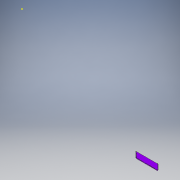
# Autodesk Inventor part: BaseBandAmp_Top_SolderMaskLower
Saved by Autodesk Inventor 2018 (Build 220112000, 112)
## iProperties
Created: 2018-03-29
Part Number: BaseBandAmp_Top_SolderMaskLower
Material: Generic
Document SubType Name: Modeling
Designer: Eric Weeks
Density: 1 g/cm^3
Appearance: Default
Author: Eric Weeks
Autodesk Inventor part; units mm, degrees
ref_plane "YZ Plane" through (0, 0, 0) normal (1, 0, 0) x (0, 1, 0)
ref_plane "XZ Plane" through (0, 0, 0) normal (0, 1, 0) x (-1, 0, 0)
ref_plane "XY Plane" through (0, 0, 0) normal (0, 0, 1) x (1, 0, 0)
sketch "Sketch1" plane through (0, 0, 0) normal (0, 0, 1) x (1, 0, 0)
  circle A0 centre (3267.7354, -2038.7056) radius 4.8387 projected
  circle A1 centre (3267.7354, -2038.7056) radius 4.8387 projected
  circle A2 centre (3287.0902, -2038.7056) radius 4.8387 projected
  circle A3 centre (3287.0902, -2038.7056) radius 4.8387 projected
  circle A4 centre (3306.445, -2038.7056) radius 4.8387 projected
  circle A5 centre (3306.445, -2038.7056) radius 4.8387 projected
  circle A6 centre (3325.7998, -2038.7056) radius 4.8387 projected
  circle A7 centre (3325.7998, -2038.7056) radius 4.8387 projected
  circle A8 centre (3345.1546, -2038.7056) radius 4.8387 projected
  circle A9 centre (3345.1546, -2038.7056) radius 4.8387 projected
  circle A10 centre (3364.5094, -2038.7056) radius 4.8387 projected
  circle A11 centre (3364.5094, -2038.7056) radius 4.8387 projected
  circle A12 centre (3383.8642, -2038.7056) radius 4.8387 projected
  circle A13 centre (3383.8642, -2038.7056) radius 4.8387 projected
  line L0 (3864.5338, -2031.6901) -> (3864.5338, -2031.8324) projected
  line L1 (3864.5338, -2031.8324) -> (3862.959, -2040.7808) projected
  line L2 (3862.959, -2040.7808) -> (3862.7558, -2041.3066) projected
  line L3 (3862.7558, -2041.3066) -> (3858.5648, -2048.5583) projected
  line L4 (3858.5648, -2048.5583) -> (3858.2092, -2048.9875) projected
  line L5 (3858.2092, -2048.9875) -> (3851.783, -2054.3698) projected
  line L6 (3851.783, -2054.3698) -> (3851.5544, -2054.5146) projected
  line L7 (3851.5544, -2054.5146) -> (3851.3004, -2054.6492) projected
  line L8 (3851.3004, -2054.6492) -> (3843.0962, -2057.6362) projected
  line L9 (3843.0962, -2057.6362) -> (3842.893, -2057.6718) projected
  line L10 (3842.893, -2057.6718) -> (3842.6898, -2057.7277) projected
  line L11 (3842.6898, -2057.7277) -> (3838.4988, -2058.096) projected
  line L12 (3838.4988, -2058.096) -> (3838.4226, -2058.0883) projected
  line L13 (3838.4226, -2058.0883) -> (3838.3464, -2058.101) projected
  line L14 (3838.3464, -2058.101) -> (3258.7692, -2058.101) projected
  line L15 (3258.7692, -2058.101) -> (3258.6168, -2058.0756) projected
  line L16 (3258.6168, -2058.0756) -> (3258.4898, -2058.0756) projected
  line L17 (3258.4898, -2058.0756) -> (3249.5236, -2056.4983) projected
  line L18 (3249.5236, -2056.4983) -> (3249.4982, -2056.4881) projected
  line L19 (3249.4982, -2056.4881) -> (3249.0156, -2056.3078) projected
  line L20 (3249.0156, -2056.3078) -> (3241.7512, -2052.1193) projected
  line L21 (3241.7512, -2052.1193) -> (3241.3194, -2051.7612) projected
  line L22 (3241.3194, -2051.7612) -> (3235.9346, -2045.3452) projected
  line L23 (3235.9346, -2045.3452) -> (3235.7568, -2045.0378) projected
  line L24 (3235.7568, -2045.0378) -> (3235.6552, -2044.86) projected
  line L25 (3235.6552, -2044.86) -> (3232.6834, -2036.6558) projected
  line L26 (3232.6834, -2036.6558) -> (3232.6326, -2036.4475) projected
  line L27 (3232.6326, -2036.4475) -> (3232.5818, -2036.2443) projected
  line L28 (3232.5818, -2036.2443) -> (3232.2262, -2032.0432) projected
  line L29 (3232.2262, -2032.0432) -> (3232.2008, -1884.2664) projected
  line L30 (3232.2008, -1884.2664) -> (3864.5592, -1884.2664) projected
  line L31 (3864.5592, -1884.2664) -> (3864.5592, -2031.553) projected
  line L32 (3864.5592, -2031.553) -> (3864.5338, -2031.6901) projected
  line L33 (3232.2262, -2032.0432) -> (3232.2262, -2031.9746) projected
  line L34 (3232.2262, -2031.9746) -> (3232.2008, -2031.9035) projected
  circle A14 centre (3248.3806, -2038.7056) radius 4.8387 projected
  circle A15 centre (3248.3806, -2038.7056) radius 4.8387 projected
  circle A16 centre (3248.3806, -2022.5766) radius 4.8387 projected
  circle A17 centre (3248.3806, -2022.5766) radius 4.8387 projected
  circle A18 centre (3248.3806, -2006.4476) radius 4.8387 projected
  circle A19 centre (3248.3806, -2006.4476) radius 4.8387 projected
  circle A20 centre (3248.3806, -1987.0928) radius 4.8387 projected
  circle A21 centre (3248.3806, -1987.0928) radius 4.8387 projected
  circle A22 centre (3848.3794, -1999.996) radius 4.8387 projected
  circle A23 centre (3848.3794, -1980.6412) radius 4.8387 projected
  circle A24 centre (3848.3794, -1980.6412) radius 4.8387 projected
  circle A25 centre (3848.3794, -1961.2864) radius 4.8387 projected
  circle A26 centre (3848.3794, -1961.2864) radius 4.8387 projected
  circle A27 centre (3848.3794, -1941.9316) radius 4.8387 projected
  circle A28 centre (3848.3794, -1941.9316) radius 4.8387 projected
  circle A29 centre (3848.3794, -1922.5768) radius 4.8387 projected
  circle A30 centre (3848.3794, -1922.5768) radius 4.8387 projected
  circle A31 centre (3848.3794, -1903.222) radius 4.8387 projected
  circle A32 centre (3848.3794, -1903.222) radius 4.8387 projected
  circle A33 centre (3848.3794, -1883.8672) radius 4.8387 projected
  circle A34 centre (3848.3794, -1883.8672) radius 4.8387 projected
  circle A35 centre (3848.3794, -1999.996) radius 4.8387 projected
  circle A36 centre (3248.3806, -1967.738) radius 4.8387 projected
  circle A37 centre (3248.3806, -1967.738) radius 4.8387 projected
  circle A38 centre (3248.3806, -1948.3832) radius 4.8387 projected
  circle A39 centre (3248.3806, -1948.3832) radius 4.8387 projected
  circle A40 centre (3248.3806, -1929.0284) radius 4.8387 projected
  circle A41 centre (3248.3806, -1909.6736) radius 4.8387 projected
  circle A42 centre (3248.3806, -1909.6736) radius 4.8387 projected
  circle A43 centre (3248.3806, -1890.3188) radius 4.8387 projected
  circle A44 centre (3248.3806, -1890.3188) radius 4.8387 projected
  circle A45 centre (3248.3806, -1929.0284) radius 4.8387 projected
  circle A46 centre (3558.0574, -2038.7056) radius 4.8387 projected
  circle A47 centre (3577.4122, -2038.7056) radius 4.8387 projected
  circle A48 centre (3596.767, -2038.7056) radius 4.8387 projected
  circle A49 centre (3616.1218, -2038.7056) radius 4.8387 projected
  circle A50 centre (3635.4766, -2038.7056) radius 4.8387 projected
  circle A51 centre (3654.8314, -2038.7056) radius 4.8387 projected
  circle A52 centre (3674.1862, -2038.7056) radius 4.8387 projected
  circle A53 centre (3693.541, -2038.7056) radius 4.8387 projected
  circle A54 centre (3712.8958, -2038.7056) radius 4.8387 projected
  circle A55 centre (3693.541, -2038.7056) radius 4.8387 projected
  circle A56 centre (3674.1862, -2038.7056) radius 4.8387 projected
  circle A57 centre (3654.8314, -2038.7056) radius 4.8387 projected
  circle A58 centre (3635.4766, -2038.7056) radius 4.8387 projected
  circle A59 centre (3616.1218, -2038.7056) radius 4.8387 projected
  circle A60 centre (3596.767, -2038.7056) radius 4.8387 projected
  circle A61 centre (3577.4122, -2038.7056) radius 4.8387 projected
  circle A62 centre (3558.0574, -2038.7056) radius 4.8387 projected
  circle A63 centre (3712.8958, -2038.7056) radius 4.8387 projected
  circle A64 centre (3848.3794, -2019.3508) radius 4.8387 projected
  circle A65 centre (3848.3794, -2019.3508) radius 4.8387 projected
  circle A66 centre (3732.2506, -2038.7056) radius 4.8387 projected
  circle A67 centre (3732.2506, -2038.7056) radius 4.8387 projected
  circle A68 centre (3751.6054, -2038.7056) radius 4.8387 projected
  circle A69 centre (3751.6054, -2038.7056) radius 4.8387 projected
  circle A70 centre (3770.9602, -2038.7056) radius 4.8387 projected
  circle A71 centre (3770.9602, -2038.7056) radius 4.8387 projected
  circle A72 centre (3790.315, -2038.7056) radius 4.8387 projected
  circle A73 centre (3790.315, -2038.7056) radius 4.8387 projected
  circle A74 centre (3809.6698, -2038.7056) radius 4.8387 projected
  circle A75 centre (3809.6698, -2038.7056) radius 4.8387 projected
  circle A76 centre (3829.0246, -2038.7056) radius 4.8387 projected
  circle A77 centre (3829.0246, -2038.7056) radius 4.8387 projected
  circle A78 centre (3848.3794, -2038.7056) radius 4.8387 projected
  circle A79 centre (3848.3794, -2038.7056) radius 4.8387 projected
  circle A80 centre (3403.219, -2038.7056) radius 4.8387 projected
  circle A81 centre (3403.219, -2038.7056) radius 4.8387 projected
  circle A82 centre (3422.5738, -2038.7056) radius 4.8387 projected
  circle A83 centre (3441.9286, -2038.7056) radius 4.8387 projected
  circle A84 centre (3441.9286, -2038.7056) radius 4.8387 projected
  circle A85 centre (3461.2834, -2038.7056) radius 4.8387 projected
  circle A86 centre (3461.2834, -2038.7056) radius 4.8387 projected
  circle A87 centre (3480.6382, -2038.7056) radius 4.8387 projected
  circle A88 centre (3480.6382, -2038.7056) radius 4.8387 projected
  circle A89 centre (3499.993, -2038.7056) radius 4.8387 projected
  circle A90 centre (3499.993, -2038.7056) radius 4.8387 projected
  circle A91 centre (3519.3478, -2038.7056) radius 4.8387 projected
  circle A92 centre (3519.3478, -2038.7056) radius 4.8387 projected
  circle A93 centre (3538.7026, -2038.7056) radius 4.8387 projected
  circle A94 centre (3538.7026, -2038.7056) radius 4.8387 projected
  circle A95 centre (3422.5738, -2038.7056) radius 4.8387 projected
  point P0 (0, 0)
extrude "Extrusion1" add sketch "Sketch1" along normal blind 0.0025 contours L0 L1 L2 L3 L4 L5 L6 L7 L8 L9 L10 L11 L12 L13 L14 L15 L16 L17 L18 L19 L20 L21 L22 L23 L24 L25 L26 L27 L28 L29 L30 A33 L31 L32 | A33 L30 picked at (3848.3794, -1885.7462)
sketch "Sketch2" plane through (0, 0, 0.0025) normal (0, 0, 1) x (1, 0, 0)
  point P0 (0, 0)
sketch "Sketch3" plane through (0, 0, 0.0025) normal (0, 0, 1) x (1, 0, 0)
  point P0 (0, 0)
body "Solid1"
